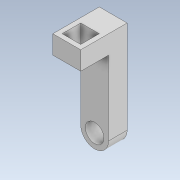
# Autodesk Inventor part: 零件2
Saved by Autodesk Inventor 2022 (Build 260153000, 153)
## iProperties
Created: 2023-04-20
Part Number: 零件2
Material: 一般
Document SubType Name: Modeling
Designer: Johnny Jou
Density: 1 g/cm^3
Appearance: 預設
Author: Johnny Jou
Autodesk Inventor part; units mm, degrees
ref_plane "YZ Plane" through (0, 0, 0) normal (1, 0, 0) x (0, 1, 0)
ref_plane "XZ Plane" through (0, 0, 0) normal (0, 1, 0) x (-1, 0, 0)
ref_plane "XY Plane" through (0, 0, 0) normal (0, 0, 1) x (1, 0, 0)
sketch "草圖1" plane through (0, 0, 0) normal (0, 0, 1) x (1, 0, 0)
  circle A0 centre (0, 0) radius 5
  line L0 (0, 0) -> (0, 50) construction
  line L1 (-7.5, 0) -> (-7.5, 50)
  line L2 (7.5, 50) -> (7.5, 0)
  arc A1 (-7.5, 0) -> (7.5, 0) centre (0, 0) ccw
  arc A2 (7.5, 50) -> (-7.5, 50) centre (0, 50) ccw
  line L3 (-7.5, 50) -> (7.5, 50)
  point P0 (0, 25)
  dimension "d0" = 10
  dimension "d1" = 15
  dimension "d2" = 50
  constraints: 10 end point, 4 point on circle, 4 tangent, 3 centre point, 1 coincident, 1 horizontal, 1 midpoint, 1 parallel, 1 vertical
  measures "d0" diameter of A0
  measures "d1" distance between parallel lines of L2 L1
  measures "d2" distance of L0.start L0.end
extrude "擠出1" add sketch "草圖1" along normal blind 10 contours L1 L3 L2 A1
sketch "草圖2" plane through (-7.5, 50, 0) normal (0, 1, 0) x (1, 0, 0)
  line L0 (15, -10) -> (0, -10) projected
  line L1 (0, -10) -> (15, -10)
  line L2 (15, -10) -> (15, -25)
  line L3 (15, -25) -> (0, -25)
  line L4 (0, -25) -> (0, -10)
  line L5 (2.5, -22.5) -> (12.5, -22.5)
  line L6 (12.5, -22.5) -> (12.5, -12.5)
  line L7 (12.5, -12.5) -> (2.5, -12.5)
  line L8 (2.5, -12.5) -> (2.5, -22.5)
  point P0 (7.5, 0)
  dimension "d5" = 10
  dimension "d6" = 10
  dimension "d7" = 2.5
  dimension "d8" = 2.5
  dimension "d9" = 15
  dimension "d10" = 15
  constraints: 16 end point, 4 parallel, 2 horizontal, 2 perpendicular
  measures "d5" distance of L5.start L5.end
  measures "d6" distance of L7.end L5.start
  measures "d7" distance between parallel lines of L4 L8
  measures "d8" distance between parallel lines of L0 L7
  measures "d9" distance between parallel lines of L0 L3
  measures "d10" distance between parallel lines of L4 L2
extrude "擠出2" add sketch "草圖2" against normal blind 10
